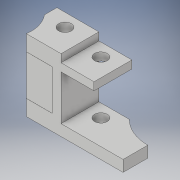
# Autodesk Inventor part: ServoBase
Saved by Autodesk Inventor 2018 (Build 220112000, 112)
## iProperties
Created: 2019-06-12
Part Number: ServoBase
Material: Generic
Document SubType Name: Modeling
Designer: anirudh
Density: 1 g/cm^3
Appearance: Default
Author: anirudh
Autodesk Inventor part; units mm, degrees
ref_plane "YZ Plane" through (0, 0, 0) normal (1, 0, 0) x (0, 1, 0)
ref_plane "XZ Plane" through (0, 0, 0) normal (0, 1, 0) x (-1, 0, 0)
ref_plane "XY Plane" through (0, 0, 0) normal (0, 0, 1) x (1, 0, 0)
sketch "Sketch1" plane through (0, 0, 0) normal (0, 1, 0) x (-1, 0, 0)
  arc A0 (-17.5636, 5.8132) -> (-8.5833, 9.5329) centre (-17.5636, 18.5132) ccw
  arc A1 (-17.5636, 5.8132) -> (-8.5833, 9.5329) centre (-17.5636, 18.5132) ccw
  arc A2 (-8.5833, -9.3366) -> (-17.5636, -5.6168) centre (-17.5636, -18.3168) ccw
  arc A3 (-8.5833, -9.3366) -> (-17.5636, -5.6168) centre (-17.5636, -18.3168) ccw
  line L0 (-17.5636, 5.8132) -> (-17.5636, -5.6168)
  line L1 (-8.5833, 9.5329) -> (11.8765, 9.5329)
  line L2 (-8.5833, -9.3366) -> (11.1934, -9.3366)
  arc A4 (11.8765, 6.0101) -> (11.8765, -5.8137) centre (18.8929, 0.0982) ccw
  line L3 (11.8765, -9.3366) -> (11.1934, -9.3366)
  line L4 (11.8765, 9.5329) -> (11.8765, 6.0101)
  line L5 (11.8765, -5.8137) -> (11.8765, -9.3366)
  circle A5 centre (5.9079, 5.8536) radius 1.8
  circle A6 centre (5.9079, 5.8536) radius 1.8
  circle A7 centre (-4.2521, 5.8536) radius 1.8
  circle A8 centre (-4.2521, 5.8536) radius 1.8
  circle A9 centre (5.9079, -5.6573) radius 1.8
  circle A10 centre (5.9079, -5.6573) radius 1.8
  circle A11 centre (-4.2521, -5.6573) radius 1.8
  circle A12 centre (-4.2521, -5.6573) radius 1.8
  point P0 (12.4052, 6.5859)
  constraints: 13 centre point, 12 end point, 11 point on circle, 5 coincident, 1 collinear
extrude "Extrusion1" add sketch "Sketch1" along normal blind 4.445
sketch "Sketch2" plane through (0, 4.445, 0) normal (0, 1, 0) x (1, 0, 0)
  line L0 (-11.8765, -9.5329) -> (8.5833, -9.5329) projected
  line L1 (8.5833, 9.3366) -> (-11.8765, 9.3366) projected
  line L2 (0, -9.5329) -> (-2.54, -9.5329)
  line L3 (-2.54, 9.3366) -> (0, 9.3366)
  line L4 (0, 9.3366) -> (0, -9.5329)
  line L5 (-2.54, -1.3682) -> (-9.8062, -1.3682)
  line L6 (-2.54, 1.1718) -> (-9.8062, 1.1718)
  arc A0 (-11.8765, -6.0101) -> (-11.8765, 5.8137) centre (-18.8929, -0.0982) ccw projected
  arc A1 (-9.8062, -1.3682) -> (-9.8062, 1.1718) centre (-18.8929, -0.0982) ccw
  line L7 (-2.54, -9.5329) -> (-2.54, -1.3682)
  line L8 (-2.54, 1.1718) -> (-2.54, 9.3366)
  point P0 (0, 0)
  dimension "d2" = 2.54
  constraints: 14 end point, 4 point on circle, 3 parallel, 2 perpendicular, 2 point on line, 1 centre point, 1 horizontal
  measures "d2" distance of L3.start L3.end
extrude "Extrusion2" add sketch "Sketch2" along normal blind 11.43
sketch "Sketch3" plane through (0, 4.445, 0) normal (0, 1, 0) x (1, 0, 0)
  line L0 (0, -11.1934) -> (18.2988, -11.1934)
  line L1 (18.2988, -11.1934) -> (18.2988, 11.7125)
  line L2 (18.2988, 11.7125) -> (0, 11.7125)
  line L3 (0, 11.7125) -> (0, -11.1934)
  point P0 (0, 0)
  constraints: 8 end point, 2 parallel, 1 horizontal, 1 perpendicular
extrude "Extrusion3" cut sketch "Sketch3" against normal blind 1.27
sketch "Sketch4" plane through (0, 15.875, 0) normal (0, 1, 0) x (1, 0, 0)
  arc A0 (20.271, 9.3366) -> (20.3081, -9.5329) centre (70.2056, 0) ccw
  line L0 (8.5833, -9.5329) -> (0, -9.5329) projected
  line L1 (-11.8765, -6.0101) -> (-11.8765, -9.5329) projected
  line L2 (7.4252, -9.5329) -> (-11.8765, -9.5329)
  line L3 (-11.8765, -9.5329) -> (-11.8765, -6.0101)
  arc A1 (-11.8765, -6.0101) -> (-11.8765, 5.8137) centre (-18.8929, -0.0982) ccw projected
  line L4 (-11.8765, 9.3366) -> (-11.8765, 5.8137) projected
  line L5 (-11.8765, 5.8137) -> (-11.8765, 9.3366)
  line L6 (-11.8765, 9.3366) -> (7.3957, 9.3366)
  line L7 (0, 9.3366) -> (8.5833, 9.3366) projected
  arc A2 (-11.8765, -6.0101) -> (-11.8765, 5.8137) centre (-18.8929, -0.0982) ccw
  line L8 (-11.8765, -9.5329) -> (8.5833, -9.5329) projected
  line L9 (-11.8765, -9.5329) -> (20.3081, -9.5329)
  line L10 (8.5833, 9.3366) -> (-11.8765, 9.3366) projected
  line L11 (-11.8765, 9.3366) -> (20.271, 9.3366)
  circle A3 centre (-5.9079, -5.8536) radius 1.8 projected
  circle A4 centre (-5.9079, -5.8536) radius 1.8
  circle A5 centre (-5.9079, 5.6573) radius 1.8 projected
  circle A6 centre (-5.9079, 5.6573) radius 1.8
  circle A7 centre (4.2521, -5.8536) radius 1.8 projected
  circle A8 centre (4.2521, -5.8536) radius 1.8
  circle A9 centre (4.2521, 5.6573) radius 1.8 projected
  circle A10 centre (4.2521, 5.6573) radius 1.8
  circle A11 centre (14.4121, -0.0982) radius 1.8
  point P0 (0, 0)
  dimension "d10" = 101.6
  dimension "d13" = 3.6
  constraints: 12 end point, 7 centre point, 5 point on circle, 4 coincident, 4 point on line, 2 collinear, 1 horizontal, 1 perpendicular
  measures "d10" diameter of A0
  measures "d13" diameter of A11
extrude "Extrusion4" add sketch "Sketch4" along normal blind 4.445
sketch "Sketch5" plane through (0, 20.32, 0) normal (0, 1, 0) x (1, 0, 0)
  line L0 (0, -9.5329) -> (20.3081, -9.5329) projected
  line L1 (20.3081, -9.5329) -> (0, -9.5329)
  line L2 (0, -9.5329) -> (0, 9.3366) projected
  line L3 (0, -9.5329) -> (0, 9.3366)
  line L4 (20.271, 9.3366) -> (0, 9.3366) projected
  line L5 (0, 9.3366) -> (20.271, 9.3366)
  arc A0 (20.271, 9.3366) -> (20.3081, -9.5329) centre (70.2056, 0) ccw
  circle A1 centre (4.2521, -5.8536) radius 1.8 projected
  circle A2 centre (4.2521, -5.8536) radius 1.8
  circle A3 centre (4.2521, 5.6573) radius 1.8 projected
  circle A4 centre (4.2521, 5.6573) radius 1.8
  circle A5 centre (14.4121, -0.0982) radius 1.8 projected
  circle A6 centre (14.4121, -0.0982) radius 1.8
  point P0 (0, 0)
  constraints: 6 end point, 4 centre point, 3 coincident, 3 collinear, 3 point on circle
extrude "Extrusion5" cut sketch "Sketch5" against normal blind 2.2225
sketch "Sketch9" plane through (-11.8765, 0, 9.5329) normal (0, 0, 1) x (1, 0, 0)
  line L0 (-6.6056, 25.3261) -> (40.6741, 25.3261)
  line L1 (40.6741, 25.3261) -> (40.6741, -4.6288)
  line L2 (40.6741, -4.6288) -> (-6.6056, -4.6288)
  line L3 (-6.6056, -4.6288) -> (-6.6056, 25.3261)
  point P0 (11.8765, 0)
  constraints: 8 end point, 2 parallel, 1 horizontal, 1 perpendicular
extrude "Extrusion7" cut sketch "Sketch9" against normal blind 8.1534
sketch "Sketch10" plane through (0, 18.0975, 0) normal (0, 1, 0) x (1, 0, 0)
  circle A0 centre (4.2521, 5.6573) radius 1.8 projected
  line L0 (0, -1.3795) -> (0, 9.3366) projected
  line L1 (9.3321, 9.9549) -> (21.2421, 9.9549)
  line L2 (21.2421, 9.9549) -> (21.2421, -3.3791)
  line L3 (21.2421, -3.3791) -> (9.3321, -3.3791)
  line L4 (9.3321, -3.3791) -> (9.3321, 9.9549)
  point P0 (0, 0)
  constraints: 8 end point, 2 parallel, 1 horizontal, 1 perpendicular
extrude "Extrusion8" cut sketch "Sketch10" against normal blind 8.1534 contours L1 L2 L3 L4
body "Solid1"
